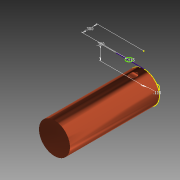
# Autodesk Inventor part: Copper
Saved by Autodesk Inventor 2014 (Build 180170000, 170)
## iProperties
Created: 2014-06-10
Part Number: Copper
Material: Generic
Document SubType Name: Modeling
Designer: Nabeel
Density: 1 g/cm^3
Appearance: Blue-Yellow
Author: Nabeel
Autodesk Inventor part; units mm, degrees
ref_plane "YZ Plane" through (0, 0, 0) normal (1, 0, 0) x (0, 1, 0)
ref_plane "XY Plane" through (0, 0, 0) normal (0, 0, 1) x (1, 0, 0)
sketch "Sketch1" plane through (0, 0, 0) normal (0, 0, 1) x (1, 0, 0)
  circle A0 centre (0, 0) radius 7.9375
  dimension "d0" = 15.875
  constraints: 1 centre point, 1 coincident
  measures "d0" diameter of A0
extrude "Extrusion1" add sketch "Sketch1" along normal blind 45.72
ref_plane "Work Plane2" through (0, 15.875, 0) normal (0, 1, 0) x (-1, 0, 0)
sketch "Sketch4" plane through (0, 15.875, 0) normal (0, 1, 0) x (-1, 0, 0)
  circle A0 centre (0, 7.62) radius 1.4605
  point P0 (0, 0)
  dimension "d6" = 2.921
  dimension "d7" = 7.62
  constraints: 1 centre point
  measures "d6" diameter of A0
  measures "d7" distance of point (0, 0) A0.centre
sketch "Sketch5" plane through (0, 0, 0) normal (0, 0, -1) x (-1, 0, 0)
  circle A0 centre (0, 0) radius 7.9375 projected
  circle A1 centre (0, 0.3175) radius 1.4605
  line L0 (0, 7.9375) -> (14.2875, 7.9375)
  dimension "d8" = 2.921
  dimension "d9" = 7.62
  constraints: 2 end point, 2 horizontal, 1 centre point, 1 vertical alignment, 1 other
  measures "d8" diameter of A1
  measures "d9" distance from line of A1.centre L0
ref_plane "Work Plane3" through (0, 7.9375, 0) normal (0, 0.7071, 0.7071) x (-1, 0, 0)
sketch "Sketch6" plane through (0, 7.9375, 0) normal (0, 0.7071, 0.7071) x (-1, 0, 0)
  circle A0 centre (0, 3.9683) radius 1.5875
  point P0 (0, 5.6127)
  dimension "d11" = 3.175
  constraints: 1 centre point
  measures "d11" diameter of A0
extrude "Extrusion2" add sketch "Sketch6" along normal mid plane 25.4
sketch "Sketch7" plane through (0, -3.8488, -6.1742) normal (0, -0.7071, -0.7071) x (-1, 0, 0)
  circle A0 centre (0, 0) radius 1.5875 projected
  circle A1 centre (0, 0) radius 1.5875 projected
  point P0 (0, -1.6443)
hole "Hole1" at (-0.0004, -3.8478, -6.1752) direction (0, 0.7071, 0.7071) diameter 3.302 depth 25.4 tip angle 118
body "Solid1"
